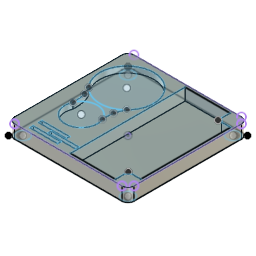
CarHolder_okey_token (Autodesk Fusion 360 design; units mm, degrees)
part number: 2025-10-28-13-39-14-687
Autodesk Fusion 360 part; units mm, degrees
sketch "Base late" plane through (0, 0, 0) normal (0, 0, 1) x (1, 0, 0)
  line L0 (-45, 50) -> (45, 50)
  line L1 (50, 45) -> (50, -45)
  line L2 (45, -50) -> (-45, -50)
  line L3 (-50, -45) -> (-50, 45)
  arc A0 (-45, 50) -> (-50, 45) centre (-45, 45) ccw
  arc A1 (50, 45) -> (45, 50) centre (45, 45) ccw
  arc A2 (45, -50) -> (50, -45) centre (45, -45) ccw
  arc A3 (-50, -45) -> (-45, -50) centre (-45, -45) ccw
  point P0 (-50, 50)
  point P1 (50, 50)
  point P2 (-50, -50)
  dimension "d1" = 100
  dimension "d2" = 100
  dimension "d3" = 50
  dimension "d4" = 50
  dimension "d5" = 5
  dimension "d6" = 5
  constraint horizontal L0
  constraint vertical L1
  constraint horizontal L2
  constraint vertical L3
  constraint coincident P0 L0
  constraint coincident P0 L3
  constraint tangent L0 A0
  constraint tangent L3 A0
  constraint coincident P1 L0
  constraint coincident P1 L1
  constraint tangent L0 A1
  constraint tangent L1 A1
  constraint tangent L1 A2
  constraint tangent L2 A2
  constraint equal A1 A2
  constraint coincident P2 L2
  constraint coincident P2 L3
  constraint tangent L2 A3
  constraint tangent L3 A3
  constraint equal A1 A3
  measures "d1" distance of P0 P2
  measures "d2" distance of P0 P1
  measures "d3" distance of origin L0
  measures "d4" distance of origin L3
  measures "d5" radius of A0
  measures "d6" radius of A1
sketch "Remote" plane through (0, 0, 0) normal (0, 0, 1) x (1, 0, 0)
  circle A0 through (-1.5, 23, 11) (-35.25, 42.4856, 11) (-35.25, 3.5144, 11)
  circle A1 through (-10.3377, -15.2955, 11) (-30.5877, -3.6041, 11) (-30.5877, -26.9868, 11)
  spline S0 degree 5 poles (-8.1085, 7.0718, 11) (-8.2864, 6.7594, 11) (-8.6325, 6.132, 11) (-9.1223, 5.1832, 11) (-9.7153, 3.9022, 11) (-10.3501, 2.2728, 11) (-10.8688, 0.6127, 11) (-11.2624, -1.0805, 11) (-11.5261, -2.8081, 11) (-11.6656, -4.5685, 11) (-11.6904, -6.3593, 11) (-11.6262, -7.8142, 11) (-11.5337, -8.9171, 11) (-11.4527, -9.6575, 11) (-11.4074, -10.029, 11) knots 0 0 0 0 0 0 0.1 0.2 0.3 0.4 0.5 0.6 0.7 0.8 0.9 1 1 1 1 1 1
  spline S1 degree 5 poles (-40.2768, 7.4657, 11) (-40.1034, 7.2246, 11) (-39.765, 6.7327, 11) (-39.2827, 5.9659, 11) (-38.6908, 4.8843, 11) (-38.0418, 3.4274, 11) (-37.4904, 1.8578, 11) (-37.0427, 0.1687, 11) (-36.6982, -1.6396, 11) (-36.4496, -3.5585, 11) (-36.2881, -5.578, 11) (-36.2221, -7.2666, 11) (-36.2059, -8.5714, 11) (-36.2096, -9.458, 11) (-36.215, -9.9055, 11) knots 0 0 0 0 0 0 0.1 0.2 0.3 0.4 0.5 0.6 0.7 0.8 0.9 1 1 1 1 1 1
  point P0 (-11.215, -1.0119)
  point P1 (-37.2605, 0.9264)
  dimension "d7" = 45
  dimension "d8" = 27
extrude "Extrude1" add sketch "Base late" along normal blind 11
extrude "Extrude2" cut sketch "Remote" against normal blind 5 contours A0 | A0 A1 S0 S1 | A1 in plane through (0, 0, 11) normal (0, 0, 1)
sketch "coins" plane through (0, 0, 11) normal (0, 0, 1) x (-1, 0, 0)
  spline S0 degree 5 poles (36.215, 9.9055) (36.2096, 9.458) (36.2059, 8.5714) (36.2221, 7.2666) (36.2881, 5.578) (36.4496, 3.5585) (36.6982, 1.6396) (37.0427, -0.1687) (37.4904, -1.8578) (38.0418, -3.4274) (38.6908, -4.8843) (39.2827, -5.9659) (39.765, -6.7327) (40.1034, -7.2246) (40.2768, -7.4657) knots -1 -1 -1 -1 -1 -1 -0.9 -0.8 -0.7 -0.6 -0.5 -0.4 -0.3 -0.2 -0.1 0 0 0 0 0 0
  arc A0 (8.1085, -7.0718) -> (40.2768, -7.4657) centre (24, -23) ccw
  spline S1 degree 5 poles (8.1085, -7.0718) (8.2864, -6.7594) (8.6325, -6.132) (9.1223, -5.1832) (9.7153, -3.9022) (10.3501, -2.2728) (10.8688, -0.6127) (11.2624, 1.0805) (11.5261, 2.8081) (11.6656, 4.5685) (11.6904, 6.3593) (11.6262, 7.8142) (11.5337, 8.9171) (11.4527, 9.6575) (11.4074, 10.029) knots 0 0 0 0 0 0 0.1 0.2 0.3 0.4 0.5 0.6 0.7 0.8 0.9 1 1 1 1 1 1
  arc A1 (36.215, 9.9055) -> (11.4074, 10.029) centre (23.8377, 15.2955) ccw
  arc A2 (45, -50) -> (50, -45) centre (45, -45) ccw
  line L0 (50, -45) -> (50, 45)
  arc A3 (50, 45) -> (45, 50) centre (45, 45) ccw
  line L1 (45, 50) -> (-45, 50)
  arc A4 (-45, 50) -> (-50, 45) centre (-45, 45) ccw
  line L2 (-50, 45) -> (-50, -45)
  arc A5 (-50, -45) -> (-45, -50) centre (-45, -45) ccw
  line L3 (-45, -50) -> (45, -50)
  line L4 (35.6994, 36.2265) -> (12.6994, 36.2265)
  line L5 (12.6994, 36.2265) -> (12.6994, 38.9265)
  line L6 (12.6994, 38.9265) -> (35.6994, 38.9265)
  line L7 (35.6994, 38.9265) -> (35.6994, 36.2265)
  line L8 (24.1994, 39.9265) -> (1.1994, 39.9265)
  line L9 (1.1994, 39.9265) -> (1.1994, 42.6265)
  line L10 (1.1994, 42.6265) -> (24.1994, 42.6265)
  line L11 (24.1994, 42.6265) -> (24.1994, 39.9265)
  line L12 (12.6347, 46.3265) -> (35.6347, 46.3265)
  line L13 (35.6347, 43.6265) -> (12.6347, 43.6265)
  line L14 (12.6347, 43.6265) -> (12.6347, 46.3265)
  line L15 (35.6347, 46.3265) -> (35.6347, 43.6265)
  dimension "d15" = 23
  dimension "d16" = 2.7
  dimension "d17" = 23
  dimension "d18" = 2.7
  dimension "d19" = 23
  dimension "d20" = 2.7
  dimension "d21" = 1
  dimension "d22" = 1
  dimension "d23" = 11.5
  constraint horizontal L4
  constraint vertical L5
  constraint horizontal L6
  constraint vertical L7
  constraint horizontal L8
  constraint vertical L9
  constraint horizontal L10
  constraint vertical L11
  constraint horizontal L13
  constraint vertical L14
  constraint horizontal L12
  constraint vertical L15
  measures "d15" distance of L4.start L4.end
  measures "d16" distance of L4.end L5.end
  measures "d17" distance of L8.start L8.end
  measures "d18" distance of L8.end L9.end
  measures "d19" distance of L13.start L13.end
  measures "d20" distance of L13.end L12.start
  measures "d21" distance of L6 L8
  measures "d22" distance of L10 L13
  measures "d23" distance of L7 L11
extrude "Extrude3" cut sketch "coins" against normal blind 10 contours L4 L5 L6 L7 | L8 L9 L10 L11 | L12 L13 L14 L15
sketch "hole" plane through (0, 0, 11) normal (0, 0, 1) x (-1, 0, 0)
  line L0 (12.6994, 36.2265) -> (12.6994, 38.9265)
  line L1 (12.6994, 38.9265) -> (35.6994, 38.9265)
  line L2 (35.6994, 38.9265) -> (35.6994, 36.2265)
  line L3 (35.6994, 36.2265) -> (12.6994, 36.2265)
  line L4 (1.1994, 39.9265) -> (1.1994, 42.6265)
  line L5 (1.1994, 42.6265) -> (24.1994, 42.6265)
  line L6 (24.1994, 42.6265) -> (24.1994, 39.9265)
  line L7 (24.1994, 39.9265) -> (1.1994, 39.9265)
  line L8 (12.6347, 43.6265) -> (12.6347, 46.3265)
  line L9 (12.6347, 46.3265) -> (35.6347, 46.3265)
  line L10 (35.6347, 46.3265) -> (35.6347, 43.6265)
  line L11 (35.6347, 43.6265) -> (12.6347, 43.6265)
  spline S0 degree 5 poles (36.215, 9.9055) (36.2096, 9.458) (36.2059, 8.5714) (36.2221, 7.2666) (36.2881, 5.578) (36.4496, 3.5585) (36.6982, 1.6396) (37.0427, -0.1687) (37.4904, -1.8578) (38.0418, -3.4274) (38.6908, -4.8843) (39.2827, -5.9659) (39.765, -6.7327) (40.1034, -7.2246) (40.2768, -7.4657) knots -1 -1 -1 -1 -1 -1 -0.9 -0.8 -0.7 -0.6 -0.5 -0.4 -0.3 -0.2 -0.1 0 0 0 0 0 0
  arc A0 (8.1085, -7.0718) -> (40.2768, -7.4657) centre (24, -23) ccw
  spline S1 degree 5 poles (8.1085, -7.0718) (8.2864, -6.7594) (8.6325, -6.132) (9.1223, -5.1832) (9.7153, -3.9022) (10.3501, -2.2728) (10.8688, -0.6127) (11.2624, 1.0805) (11.5261, 2.8081) (11.6656, 4.5685) (11.6904, 6.3593) (11.6262, 7.8142) (11.5337, 8.9171) (11.4527, 9.6575) (11.4074, 10.029) knots 0 0 0 0 0 0 0.1 0.2 0.3 0.4 0.5 0.6 0.7 0.8 0.9 1 1 1 1 1 1
  arc A1 (36.215, 9.9055) -> (11.4074, 10.029) centre (23.8377, 15.2955) ccw
  arc A2 (45, -50) -> (50, -45) centre (45, -45) ccw
  line L12 (50, -45) -> (50, 45)
  arc A3 (50, 45) -> (45, 50) centre (45, 45) ccw
  line L13 (45, 50) -> (-45, 50)
  arc A4 (-45, 50) -> (-50, 45) centre (-45, 45) ccw
  line L14 (-50, 45) -> (-50, -45)
  arc A5 (-50, -45) -> (-45, -50) centre (-45, -45) ccw
  line L15 (-45, -50) -> (45, -50)
  line L16 (0.1496, -48) -> (-37.4819, -48)
  line L17 (-37.4819, 48) -> (0.1496, 48)
  line L18 (0.1496, 48) -> (0.1496, -48)
  line L19 (-40.4819, -37.8864) -> (-48, -37.8864)
  line L20 (-48, -37.8864) -> (-48, 37.2468)
  line L21 (-48, 37.2468) -> (-40.4819, 37.2468)
  line L22 (-37.4819, -48) -> (-37.4819, -40.8864)
  line L23 (-37.4819, 40.2468) -> (-37.4819, 48)
  line L24 (-40.4819, -37.8864) -> (-37.4819, -40.8864)
  line L25 (-40.4819, 37.2468) -> (-37.4819, 40.2468)
  line L26 (45, -50) -> (-45, -50)
  line L27 (-50, -45) -> (-50, 45)
  line L28 (-45, 50) -> (45, 50)
  point P0 (-37.4819, -37.8864)
  point P1 (-37.4819, 37.2468)
  dimension "d44" = 3
  dimension "d45" = 3
  dimension "d46" = 3
  dimension "d47" = 3
  dimension "d48" = 2
  dimension "d49" = 2
  dimension "d50" = 2
  constraint horizontal L16
  constraint vertical L22
  constraint horizontal L17
  constraint vertical L18
  constraint horizontal L19
  constraint vertical L20
  constraint horizontal L21
  constraint coincident P0 L19
  constraint coincident P0 L22
  constraint coincident P1 L21
  constraint coincident P1 L23
  measures "d44" distance of P0 L19.start
  measures "d45" distance of P0 L22.end
  measures "d46" distance of P1 L21.end
  measures "d47" distance of P1 L23.start
  measures "d48" distance of L16 L26
  measures "d49" distance of L20 L27
  measures "d50" distance of L17 L28
sketch "magnets" plane through (0, 0, 0) normal (0, 0, 1) x (1, 0, 0)
  circle A0 centre (44, -44) radius 5.1
  circle A1 centre (44, 44) radius 5.1
  circle A2 centre (-44, 44) radius 5.1
  circle A3 centre (-44, -44) radius 5.1
  dimension "d32" = 10.2
  dimension "d33" = 10.2
  dimension "d34" = 10.2
  dimension "d35" = 10.2
  measures "d32" diameter of A0
  measures "d33" diameter of A1
  measures "d34" diameter of A2
  measures "d35" diameter of A3
extrude "Extrude5" cut sketch "magnets" along normal blind 2.2 contours A0
extrude "Extrude6" cut sketch "magnets" along normal blind 2.2 contours A1
extrude "Extrude7" cut sketch "magnets" along normal blind 2.2 contours A3
extrude "Extrude8" cut sketch "magnets" along normal blind 2.2 contours A2
extrude "Extrude9" cut sketch "hole" against normal blind 10 contours L16 L17 L18 L19 L20 L21 L22 L23 L24 L25
equation "d23 = ( 23 / 2 ) * 1 mm"
equation "d45 = d44"
equation "d47 = d46"
